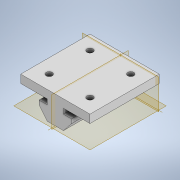
# Autodesk Inventor part: IDOM_infrared_fixture1
Saved by Autodesk Inventor 2022 (Build 260153000, 153)
## iProperties
Created: 2022-07-06
Part Number: IDOM_infrared_fixture1
Material: Generic
Document SubType Name: Modeling
Designer: dovalle
Density: 1 g/cm^3
Appearance: Default
Author: dovalle
Autodesk Inventor part; units mm, degrees
sketch "Sketch1" plane through (0, 0, 0) normal (0, 0, 1) x (1, 0, 0)
  line L0 (0, 0) -> (4, 0)
  line L1 (0, 0) -> (-4, 0)
  line L2 (-4, 7) -> (-4, 9.5)
  line L3 (4, 7) -> (4, 9.5)
  line L4 (-4, 7) -> (-8, 7)
  line L5 (4, 7) -> (8, 7)
  line L6 (-8, 7) -> (-8, 5)
  line L7 (8, 7) -> (8, 5)
  line L8 (8, 5) -> (4, 0)
  line L9 (-8, 5) -> (-4, 0)
  line L10 (-4, 9.5) -> (-15, 9.5)
  line L11 (4, 9.5) -> (15, 9.5)
  line L12 (-15, 9.5) -> (-15, 13.5)
  line L13 (-15, 13.5) -> (15, 13.5)
  line L14 (15, 13.5) -> (15, 9.5)
  dimension "d12" = 4
  constraints: 30 end point, 5 horizontal, 5 vertical, 2 perpendicular
  measures "d12" distance of L10.end L12.end
extrude "Extrusion1" add sketch "Sketch1" along normal blind 30
sketch "Sketch2" plane through (-15, 13.5, 0) normal (0, 1, 0) x (1, 0, 0)
  line L0 (0, -30) -> (11, -30) projected
  line L1 (30, 0) -> (30, -30) projected
  line L2 (30, 0) -> (0, 0) projected
  circle A0 centre (5, -5) radius 1.5
  circle A1 centre (5, -25) radius 1.5
  circle A2 centre (25, -25) radius 1.5
  circle A3 centre (25, -5) radius 1.5
  point P0 (15, 0)
  point P1 (15, -15)
  dimension "d19" = 360
  constraints: 4 centre point, 9 other
extrude "Extrusion2" cut sketch "Sketch2" against normal blind 5
sketch "Sketch3" plane through (-15, 9.5, 0) normal (0, -1, 0) x (1, 0, 0)
  line L0 (3.5, 7.5981) -> (6.5, 7.5981)
  line L1 (6.5, 7.5981) -> (8, 5)
  line L2 (8, 5) -> (6.5, 2.4019)
  line L3 (6.5, 2.4019) -> (3.5, 2.4019)
  line L4 (3.5, 2.4019) -> (2, 5)
  line L5 (2, 5) -> (3.5, 7.5981)
  line L6 (3.5, 27.5981) -> (6.5, 27.5981)
  line L7 (6.5, 27.5981) -> (8, 25)
  line L8 (8, 25) -> (6.5, 22.4019)
  line L9 (6.5, 22.4019) -> (3.5, 22.4019)
  line L10 (3.5, 22.4019) -> (2, 25)
  line L11 (2, 25) -> (3.5, 27.5981)
  line L12 (23.5, 7.5981) -> (26.5, 7.5981)
  line L13 (26.5, 7.5981) -> (28, 5)
  line L14 (28, 5) -> (26.5, 2.4019)
  line L15 (26.5, 2.4019) -> (23.5, 2.4019)
  line L16 (23.5, 2.4019) -> (22, 5)
  line L17 (22, 5) -> (23.5, 7.5981)
  line L18 (23.5, 27.5981) -> (26.5, 27.5981)
  line L19 (26.5, 27.5981) -> (28, 25)
  line L20 (28, 25) -> (26.5, 22.4019)
  line L21 (26.5, 22.4019) -> (23.5, 22.4019)
  line L22 (23.5, 22.4019) -> (22, 25)
  line L23 (22, 25) -> (23.5, 27.5981)
  point P0 (15, 0)
  dimension "d23" = 3
  dimension "d24" = 3
  dimension "d26" = 3
  dimension "d27" = 120
  dimension "d28" = 3
  dimension "d29" = 120
  dimension "d30" = 3
  dimension "d31" = 3
  dimension "d32" = 120
  dimension "d33" = 3
  dimension "d34" = 120
  dimension "d35" = 3
  dimension "d36" = 120
  dimension "d37" = 3
  dimension "d38" = 3
  dimension "d40" = 3
  dimension "d41" = 120
  dimension "d42" = 3
  dimension "d43" = 120
  dimension "d44" = 3
  dimension "d45" = 3
  dimension "d46" = 120
  dimension "d47" = 3
  dimension "d48" = 120
  dimension "d49" = 3
  dimension "d50" = 120
  constraints: 48 end point, 12 parallel, 4 horizontal
  measures "d23" distance of L0.start L0.end
  measures "d24" distance of L0.end L1.end
  measures "d26" distance of L1.end L2.end
  measures "d27" angle of L1 L2
  measures "d28" distance of L3.end L4.end
  measures "d29" angle of L3 L4
  measures "d30" distance of L6.start L6.end
  measures "d31" distance of L6.end L7.end
  measures "d32" angle of L6 L7
  measures "d33" distance of L7.end L8.end
  measures "d34" angle of L7 L8
  measures "d35" distance of L9.end L10.end
  measures "d36" angle of L9 L10
  measures "d37" distance of L17.end L12.end
  measures "d38" distance of L12.end L14.start
  measures "d40" distance of L14.start L15.start
  measures "d41" angle of L13 L14
  measures "d42" distance of L15.end L16.end
  measures "d43" angle of L15 L16
  measures "d44" distance of L23.end L18.end
  measures "d45" distance of L18.end L20.start
  measures "d46" angle of L18 L19
  measures "d47" distance of L20.start L21.start
  measures "d48" angle of L19 L20
  measures "d49" distance of L21.end L22.end
  measures "d50" angle of L21 L22
extrude "Extrusion3" cut sketch "Sketch3" against normal blind 2.2
sketch "Sketch4" plane through (0, 0, 30) normal (0, 0, 1) x (1, 0, 0)
  line L0 (-8, 7) -> (-8, 5) projected
  line L1 (-8, 5) -> (-4, 0) projected
  line L2 (-4, 0) -> (4, 0) projected
  line L3 (4, 0) -> (8, 5) projected
  line L4 (8, 5) -> (8, 7) projected
  line L5 (8, 7) -> (4, 7) projected
  line L6 (4, 7) -> (4, 9.5) projected
  line L7 (4, 9.5) -> (15, 9.5) projected
  line L8 (15, 9.5) -> (15, 13.5) projected
  line L9 (15, 13.5) -> (-15, 13.5) projected
  line L10 (-15, 13.5) -> (-15, 9.5) projected
  line L11 (-15, 9.5) -> (-4, 9.5) projected
  line L12 (-4, 9.5) -> (-4, 7) projected
  line L13 (-4, 7) -> (-8, 7) projected
  line L14 (-8, 7) -> (-8, 5) projected
  line L15 (-8, 5) -> (-4, 0) projected
  line L16 (-4, 0) -> (4, 0) projected
  line L17 (4, 0) -> (8, 5) projected
  line L18 (8, 5) -> (8, 7) projected
  line L19 (8, 7) -> (4, 7) projected
  line L20 (4, 7) -> (4, 9.5) projected
  line L21 (4, 9.5) -> (15, 9.5) projected
  line L22 (15, 9.5) -> (15, 13.5) projected
  line L23 (15, 13.5) -> (-15, 13.5) projected
  line L24 (-15, 13.5) -> (-15, 9.5) projected
  line L25 (-15, 9.5) -> (-4, 9.5) projected
  line L26 (-4, 9.5) -> (-4, 7) projected
  line L27 (-4, 7) -> (-8, 7) projected
extrude "Extrusion4" add sketch "Sketch4" along normal blind 2
sketch "Sketch5" plane through (-15, 9.5, 0) normal (-1, 0, 0) x (0, 0, 1)
  line L0 (0, 4) -> (0, 0) projected
  line L1 (0, 0) -> (32, 0) projected
  line L2 (32, 4) -> (32, 0) projected
  line L3 (0, 4) -> (32, 4) projected
  point P0 (0, -9.5)
extrude "Extrusion5" add sketch "Sketch5" along normal blind 2
sketch "Sketch6" plane through (15, 9.5, 0) normal (1, 0, 0) x (0, 0, -1)
  line L0 (0, 0) -> (0, 4) projected
  line L1 (0, 4) -> (-32, 4) projected
  line L2 (-32, 0) -> (-32, 4) projected
  line L3 (0, 0) -> (-32, 0) projected
  point P0 (0, -9.5)
extrude "Extrusion6" add sketch "Sketch6" along normal blind 2
sketch "Sketch7" plane through (0, 0, 0) normal (0, 0, -1) x (-1, 0, 0)
  line L0 (8, 7) -> (8, 5) projected
  line L1 (4, 7) -> (8, 7) projected
  line L2 (4, 9.5) -> (4, 7) projected
  line L3 (4, 9.5) -> (17, 9.5) projected
  line L4 (17, 13.5) -> (17, 9.5) projected
  line L5 (17, 13.5) -> (-17, 13.5) projected
  line L6 (-17, 9.5) -> (-17, 13.5) projected
  line L7 (-4, 9.5) -> (-17, 9.5) projected
  line L8 (-4, 7) -> (-4, 9.5) projected
  line L9 (-8, 7) -> (-4, 7) projected
  line L10 (-8, 5) -> (-8, 7) projected
  line L11 (-4, 0) -> (-8, 5) projected
  line L12 (4, 0) -> (-4, 0) projected
  line L13 (8, 5) -> (4, 0) projected
  point P0 (0, 0)
extrude "Extrusion7" add sketch "Sketch7" along normal blind 2
body "Solid1"
